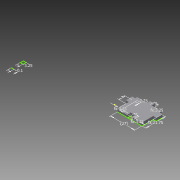
# Autodesk Inventor part: arm-servo
Saved by Autodesk Inventor 2013 (Build 170138000, 138)
## iProperties
Created: 2012-09-08
Part Number: arm-servo
Material: Generic
Document SubType Name: Modeling
Designer: frankenteddy
Density: 1 g/cm^3
Author: frankenteddy
Autodesk Inventor part; units mm, degrees
ref_plane "YZ Plane" through (0, 0, 0) normal (1, 0, 0) x (0, 1, 0)
ref_plane "XZ Plane" through (0, 0, 0) normal (0, 1, 0) x (-1, 0, 0)
ref_plane "XY Plane" through (0, 0, 0) normal (0, 0, 1) x (1, 0, 0)
sketch "Block1" plane through (0, 0, 0) normal (0, 0, 1) x (1, 0, 0)
  circle A0 centre (74.029, 24.2723) radius 1
  line L0 (49.279, 30.4723) -> (71.779, 30.4723)
  line L1 (71.779, 30.4723) -> (71.779, 18.0723)
  line L2 (71.779, 18.0723) -> (49.279, 18.0723)
  line L3 (49.279, 18.0723) -> (49.279, 30.4723)
  line L4 (49.279, 30.4723) -> (44.779, 30.4723)
  line L5 (44.779, 30.4723) -> (44.779, 18.0723)
  line L6 (44.779, 18.0723) -> (49.279, 18.0723)
  line L7 (49.279, 18.0723) -> (49.279, 30.4723)
  line L8 (71.779, 30.4723) -> (76.279, 30.4723)
  line L9 (76.279, 30.4723) -> (76.279, 18.0723)
  line L10 (76.279, 18.0723) -> (71.779, 18.0723)
  line L11 (71.779, 18.0723) -> (71.779, 30.4723)
  line L12 (44.779, 24.2723) -> (76.279, 24.2723) construction
  line L13 (47.029, 30.4723) -> (47.029, 18.0723) construction
  circle A1 centre (47.029, 24.2723) radius 1
  line L14 (74.029, 30.4723) -> (74.029, 18.0723) construction
  point P0 (60.979, 24.0984)
  dimension "d7" = 22.5
  dimension "d8" = 12.4
  dimension "d9" = 4.5
  dimension "d10" = 4.5
  dimension "d11" = 2
  dimension "d12" = 2
  measures "d7" distance of L1.end L2.end
  measures "d8" distance of L0.end L1.end
  measures "d9" distance of L6.end L5.end
  measures "d10" distance of L9.end L10.end
  measures "d11" diameter of A0
  measures "d12" diameter of A1
sketch "Sketch1" plane through (0, 0, 0) normal (0, 0, 1) x (1, 0, 0)
  line L0 (-92.7646, -8.503) -> (-89.7646, -8.503)
  line L1 (-89.7646, -8.503) -> (-89.7646, -11.753)
  line L2 (-89.7646, -11.753) -> (-92.7646, -11.753)
  line L3 (-92.7646, -11.753) -> (-92.7646, -8.503)
  line L4 (-92.7646, -21.6527) -> (-89.7646, -21.6527)
  line L5 (-89.7646, -21.6527) -> (-89.7646, -21.7527)
  line L6 (-89.7646, -21.7527) -> (-92.7646, -21.7527)
  line L7 (-92.7646, -21.7527) -> (-92.7646, -21.6527)
  line L8 (8.2387, -5.1967) -> (35.2387, -5.1967)
  line L9 (35.2387, -5.1967) -> (35.2387, 16.5533)
  line L10 (35.2387, 16.5533) -> (8.2387, 16.5533)
  line L11 (8.2387, 16.5533) -> (8.2387, -5.1967)
  line L12 (8.2387, 5.6783) -> (35.2387, 5.6783) construction
  line L13 (21.7387, 16.5533) -> (21.7387, -5.1967) construction
  line L14 (19.2387, 16.5533) -> (24.2387, 16.5533)
  line L15 (24.2387, 16.5533) -> (24.2387, 19.8033)
  line L16 (24.2387, 19.8033) -> (19.2387, 19.8033)
  line L17 (19.2387, 19.8033) -> (19.2387, 16.5533)
  line L18 (21.7387, 19.8033) -> (21.7387, 16.5533) construction
  line L19 (8.2387, 14.3033) -> (4.9887, 14.3033)
  line L20 (4.9887, 14.3033) -> (4.9887, 7.3033)
  line L21 (4.9887, 7.3033) -> (8.2387, 7.3033)
  line L22 (8.2387, 7.3033) -> (8.2387, 14.3033)
  line L23 (19.2387, -5.1967) -> (24.2387, -5.1967)
  line L24 (24.2387, -5.1967) -> (24.2387, -1.9467)
  line L25 (24.2387, -1.9467) -> (19.2387, -1.9467)
  line L26 (19.2387, -1.9467) -> (19.2387, -5.1967)
  line L27 (21.7387, -1.9467) -> (21.7387, -5.1967) construction
  line L28 (35.2387, 14.3033) -> (38.4887, 14.3033)
  line L29 (38.4887, 14.3033) -> (38.4887, 7.3033)
  line L30 (38.4887, 7.3033) -> (35.2387, 7.3033)
  line L31 (35.2387, 7.3033) -> (35.2387, 14.3033)
  point P0 (0, 0)
  dimension "d0" = 3
  dimension "mat" = 3.25
  dimension "d2" = 3
  dimension "d3" = 0.1
  dimension "d58" = 27
  dimension "d59" = 21.75
  dimension "d60" = 5
  dimension "d61" = 3.25
  dimension "d64" = 3.25
  dimension "d65" = 7
  dimension "d66" = 5
  dimension "d67" = 3.25
  dimension "d70" = 2.25
  dimension "d75" = 27
  constraints: 64 end point, 12 parallel, 8 midpoint, 6 horizontal, 6 perpendicular, 5 collinear, 4 symmetric about line
  measures "d0" distance of L1.end L3.start
  measures "mat" distance of L1.start L1.end
  measures "d2" distance of L5.end L7.start
  measures "d3" distance of L5.start L5.end
  measures "d58" distance of L10.end L9.end
  measures "d59" distance of L9.end L8.end
  measures "d60" distance of L16.end L15.end
  measures "d61" distance of L15.end L14.end
  measures "d64" distance of L21.end L20.end
  measures "d65" distance of L20.end L19.end
  measures "d66" distance of L25.end L24.end
  measures "d67" distance of L24.end L23.end
  measures "d70" distance between parallel lines of L19 L10
  measures "d75" distance between parallel lines of L9 L11
extrude "Extrusion5" add sketch "Sketch1" along normal blind 3.25 contours L11 L10 L9 L8 L24 L25 L26 | L26 L25 L24 L8 | L17 L16 L15 L10
extrude "Extrusion6" cut sketch "Sketch1" along normal blind 3.25 contours L26 L25 L24 L8
extrude "Extrusion7" add sketch "Sketch1" along normal blind 3.25 contours L21 L20 L19 L11
extrude "Extrusion8" add sketch "Sketch1" along normal blind 3.25 contours L9 L28 L29 L30
equation "\"d61\" = mat"
equation "\"d64\" = mat"
equation "\"d67\" = mat"
equation "\"d62\" = mat"
equation "\"d68\" = mat"
equation "\"d71\" = mat"
equation "\"d73\" = mat"
body "Solid4"
